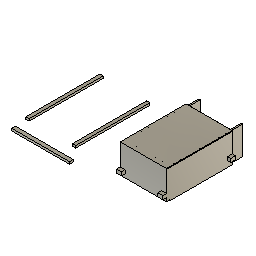
USV_cover_rect v23 (Autodesk Fusion 360 design; units mm, degrees)
Autodesk Fusion 360 part; units mm, degrees
note: some values were not read from the file. Chosen so that the rebuilt part matches the saved one: which face or edge a step refers to.
box "Primitiva de caixa1" add length 8 width 112 height 200 placed x (0, 1, 0) y (-1, 0, 0) z (0, 0, 1) at (112, 0, 0) makes body 1
box "Primitiva de caixa2" add length 100 width 3 height 200 placed x (0, 1, 0) y (-1, 0, 0) z (0, 0, 1) at (112, 0, 0) bodies 1
extrude "Extrusão1" cut 1 faces at (73.6667, 2.6667, 200) along direction (0, 0, -1) blind 100 on bodies 1 bodies 1
box "Primitiva de caixa3" add length 100 width 3 height 100 placed x (0, 1, 0) y (-1, 0, 0) z (0, 0, 1) at (3, 0, 0) bodies 1
box "Primitiva de caixa4" cut length 5 width 112 height -5 placed x (0, 1, 0) y (-1, 0, 0) z (0, 0, 1) at (112, 0, 0) bodies 1
box "Primitiva de caixa5" cut length 5 width 112 height 1 placed x (0, 1, 0) y (-1, 0, 0) z (0, 0, 1) at (112, 0, 0) bodies 1
box "Primitiva de caixa6" add length 5 width 110 height 5 placed x (0, -1, 0) y (1, 0, 0) z (0, 0, 1) at (0.5, 0, 0) bodies 1
delete_face "DeleteFace1" 6 faces at (73.8333, 0, 0.6667) (0.5, -3.3333, 2) (110.5, -3.3333, 2) (73.8333, -1.6667, 0) (73.8333, -5, 3.3333) (73.8333, -1.6667, 5) on bodies 1
box "Primitiva de caixa7" cut length 5 width 109 height 2 placed x (0, 1, 0) y (-1, 0, 0) z (0, 0, 1) at (110.5, 0, 0) bodies 1
box "Primitiva de caixa9" add length 1 width 1.5 height 109 placed x (0, 0, -1) y (0, -1, 0) z (-1, 0, 0) at (110.5, 1.5, 2) bodies 1
move_face "Deslocar faces1" offset -90 1 faces at (38.3333, 2.6667, 100) on bodies 1
sketch "Esboço10" plane through (0, 0, 0) normal (0, 0, 1) x (1, 0, 0)
sketch "Esboço11" plane through (0, 0, 0) normal (0, 0, 1) x (1, 0, 0)
box "Primitiva de caixa10" add length 10 width 3.49 height 10 placed x (0, 1, 0) y (-1, 0, 0) z (0, 0, 1) at (6.49, 95, 0) bodies 1
box "Primitiva de caixa11" add length 10 width 3.49 height 10 placed x (0, 1, 0) y (-1, 0, 0) z (0, 0, 1) at (109, 95, 0) bodies 1
extrude "Extrusão2" add 1 faces at (38.3333, 2.6667, 10) along direction (0, 0, 1) blind 60 on bodies 1 bodies 1
move_face "Deslocar faces2" offset 60 2 faces at (107.8367, 105, 23.3333) (110, 100, 46.6667) on bodies 1
move_face "Deslocar faces3" offset -60 1 faces at (106.6733, 95, 46.6667) on bodies 1
move_face "Deslocar faces4" offset 60 2 faces at (2, 100, 46.6667) (4.1633, 105, 46.6667) on bodies 1
move_face "Deslocar faces5" offset -60 1 faces at (5.3267, 95, 23.3333) on bodies 1
extrude "Extrusão3" add 2 faces at (107.8367, 165, 23.3333) (5.3267, 165, 23.3333) along direction (0, 1, 0) blind 20 on bodies 1 bodies 1
box "Primitiva de caixa12" add length 3.5 width 4 height 3.5 placed x (0, 0, 1) y (-1, 0, 0) z (0, -1, 0) at (112, 0, 6.5) bodies 1
extrude "Extrusão4" add 1 faces at (110.6667, -1.1667, 6.5) along direction (0, 0, -1) blind 0.5 on bodies 1 bodies 1
extrude "Extrusão5" add 1 faces at (108, -1.1667, 8.6667) along direction (-1, 0, 0) blind 2 on bodies 1 bodies 1
box "Primitiva de caixa13" add length 8.5 width 21 height -6 placed x (0, 0, -1) y (-1, 0, 0) z (0, 1, 0) at (21, 0, 19.5) bodies 1
extrude "Extrusão6" add 1 faces at (14, -4, 11) along direction (0, 0, 1) blind 6 on bodies 1 bodies 1
extrude "Extrusão7" cut 1 faces at (14, -4, 19.5) along direction (0, 0, 1) blind 6 on bodies 1 bodies 1
extrude "Extrusão8" cut 1 faces at (21, -4, 13.8333) along direction (-1, 0, 0) blind 9.3 on bodies 1 bodies 1
extrude "Extrusão9" add 1 faces at (108, -3.5, 7.3333) along direction (0, -1, 0) blind 2.5 on bodies 1 bodies 1
box "Primitiva de caixa14" add length 12 width 13 height 6 placed x (0, 0, 1) y (0, -1, 0) z (1, 0, 0) at (112, 160, 5) bodies 1
extrude "Extrusão10" cut 1 faces at (114, 147, 13) along direction (0, 1, 0) blind 7 on bodies 1 bodies 1
extrude "Extrusão11" cut 1 faces at (114, 158, 17) along direction (0, 0, -1) blind 8 on bodies 1 bodies 1
box "Primitiva de caixa15" add length 4 width 6 height 6 placed x (0, 0, 1) y (0, 1, 0) z (-1, 0, 0) at (0, 154, 5) bodies 1
sketch "Esboço22" plane through (112, 0, 0) normal (1, 0, 0) x (0, 1, 0)
  line L0 (160, 5) -> (154, 5)
  line L1 (154, 5) -> (154, 9)
  line L2 (154, 9) -> (160, 9)
  line L3 (160, 9) -> (160, 70)
  line L4 (160, 70) -> (0, 70)
  line L5 (0, 70) -> (0, 10)
  line L6 (0, 10) -> (-6, 10)
  line L7 (-6, 10) -> (-6, 6)
  line L8 (-6, 6) -> (0, 6)
  line L9 (0, 6) -> (0, 1)
  line L10 (0, 1) -> (5, 1)
  line L11 (5, 1) -> (5, 0)
  line L12 (5, 0) -> (160, 0)
  line L13 (160, 0) -> (160, 5)
box "Primitiva de caixa20" add length 52 width 160 height 6.5 placed x (0, 0, -1) y (0, 1, 0) z (1, 0, 0) at (112, 0, 70) bodies 1
sketch "Esboço24" plane through (0, 0, 70) normal (0, 0, 1) x (-1, 0, 0)
  line L0 (-109, -160) -> (-109, -185)
  line L1 (-109, -185) -> (-105.51, -185)
  line L2 (-105.51, -185) -> (-105.51, -155)
  line L3 (-105.51, -155) -> (-109, -155)
  line L4 (-109, -155) -> (-109, -8)
  line L5 (-109, -8) -> (-3, -8)
  line L6 (-3, -8) -> (-3, -155)
  line L7 (-3, -155) -> (-6.49, -155)
  line L8 (-6.49, -155) -> (-6.49, -185)
  line L9 (-6.49, -185) -> (-3, -185)
  line L10 (-3, -185) -> (-3, -160)
  line L11 (-3, -160) -> (0, -160)
box "Primitiva de caixa21" add length 3 width 9 height 1 placed x (0, -1, 0) y (1, 0, 0) z (0, 0, 1) at (109, 8, 70) bodies 1
extrude "Extrusão14" cut 1 faces at (115, 7, 71) along direction (0, 0, -1) blind 1 on bodies 1 bodies 1
box "Primitiva de caixa22" add length 4 width 3 height 1 placed x (0, -1, 0) y (1, 0, 0) z (0, 0, 1) at (109, 8, 70) bodies 1
box "Primitiva de caixa23" cut length 147 width 2.5 height -61 placed x (0, 1, 0) y (-1, 0, 0) z (0, 0, 1) at (114.5, 8, 70) bodies 1
extrude "Extrusão15" cut 1 faces at (118.5, 106.6667, 52.6667) along direction (-1, 0, 0) blind 6.5 on bodies 1 bodies 1
box "Primitiva de caixa24" add length 52 width 160 height -2 placed x (0, 0, -1) y (0, -1, 0) z (-1, 0, 0) at (0, 160, 70) bodies 1
move_face "MoverFace1" by (-26.3793, 1.2468, -0.5389) 1 faces at (111, 6.6667, 71) on bodies 1
extrude "Extrusão16" add 1 faces at (111, 6.6667, 70.4611) along direction (0, 0, 1) blind 2 on bodies 1 bodies 1
extrude "Extrusão17" add 1 faces at (109, 5.3333, 71.6407) along direction (-1, 0, 0) blind 109 on bodies 1 bodies 1
box "Primitiva de caixa25" cut length 147 width 2.5 height -61 placed x (0, -1, 0) y (1, 0, 0) z (0, 0, 1) at (-2.5, 155, 70) bodies 1
extrude "Extrusão18" cut 1 faces at (74.6667, 4, 70.8204) along direction (0, 1, 0) blind 4 on bodies 1 bodies 1
box "Primitiva de caixa26" add length 3 width 2 height -1 placed x (0, -1, 0) y (1, 0, 0) z (0, 0, 1) at (109, 8, 70) bodies 1
box "Primitiva de caixa27" cut length 2.5 width 106 height -52 placed x (0, -1, 0) y (1, 0, 0) z (0, 0, 1) at (3, 5, 70) bodies 1
extrude "Extrusão25" cut 1 faces at (110, 160, 29.3333) along direction (0, -1, 0) blind 3.3 on bodies 1 bodies 1
extrude "Extrusão26" cut 1 faces at (2, 160, 26.3333) along direction (0, -1, 0) blind 3.3 on bodies 1 bodies 1
extrude "Extrusão27" add 1 faces at (-2, 154, 7.6667) along direction (0, -1, 0) blind 9 on bodies 1 bodies 1
extrude "Extrusão28" add 1 faces at (114, 154, 7.6667) along direction (0, -1, 0) blind 9 on bodies 1 bodies 1
delete_face "DeleteFace2" 1 faces at (109, 3.3333, 35.3333) on bodies 1
box "Primitiva de caixa34" cut length 30 width 3.49 height -0.01 placed x (0, 1, 0) y (-1, 0, 0) z (0, 0, 1) at (109, 155, 70) bodies 1
box "Primitiva de caixa35" cut length 30 width 3.49 height -0.01 placed x (0, -1, 0) y (1, 0, 0) z (0, 0, 1) at (3, 185, 70) bodies 1
box "Primitiva de caixa36" cut length 30 width 3.49 height 0.01 placed x (0, 1, 0) y (-1, 0, 0) z (0, 0, 1) at (6.49, 155, 69.99) bodies 1
sketch "Esboço41" plane through (0, 0, 70) normal (0, 0, 1) x (-1, 0, 0)
  line L0 (-3, -8) -> (-3, -156.7)
  line L1 (-3, -156.7) -> (0, -156.7)
  line L2 (0, -156.7) -> (0, 0)
  line L3 (0, 0) -> (-112, 0)
  line L4 (-112, 0) -> (-112, -156.7)
  line L5 (-112, -156.7) -> (-109, -156.7)
  line L6 (-109, -156.7) -> (-109, -8)
  line L7 (-109, -8) -> (-3, -8)
box "Primitiva de caixa37" add length 185 width 265 height 2 placed x (0, 1, 0) y (-1, 0, 0) z (0, 0, 1) at (265, 0, 70) bodies 1
box "Primitiva de caixa38" add length 190 width 153 height 0.5 placed x (0, -1, 0) y (1, 0, 0) z (0, 0, 1) at (-153, 185, 72) separate body makes body 2
move_face "Deslocar faces6" offset 2 1 faces at (-102, 121.6667, 72) on bodies 2
extrude "Extrusão29" cut 1 faces at (-102, 121.6667, 72.5) along direction (0, 0, -1) blind 0.5 on bodies 2 bodies 2
extrude "Extrusão30" cut 1 faces at (-51, -5, 70.6667) along direction (0, 1, 0) blind 5 on bodies 2 bodies 2
box "Primitiva de caixa39" add length 165 width 418 height -2 placed x (0, -1, 0) y (1, 0, 0) z (0, 0, 1) at (-153, 0, 72) bodies 1 2
extrude "Extrusão31" cut 2 faces at (-153, -110, 70.6667) (-153, 61.6667, 70.6667) along direction (1, 0, 0) blind 150 on bodies 1 bodies 1
extrude "Extrusão32" cut 1 faces at (175.6667, -165, 70.6667) along direction (0, 1, 0) blind 95 on bodies 1 bodies 1
extrude "Extrusão33" cut 1 faces at (175.6667, -70, 70.6667) along direction (0, 1, 0) blind 65 on bodies 1 bodies 1
extrude "Extrusão34" cut 2 faces at (265, -3.3333, 70.6667) (265, 123.3333, 70.6667) along direction (-1, 0, 0) blind 150 on bodies 1 bodies 1
extrude "Extrusão35" add 2 faces at (115, 123.3333, 70.6667) (115, -3.3333, 70.6667) along direction (1, 0, 0) blind 0.441 on bodies 1 bodies 1
extrude "Extrusão36" add 2 faces at (115.441, -3.3333, 70.6667) (115.441, 123.3333, 70.6667) along direction (1, 0, 0) blind 2 on bodies 1 bodies 1
extrude "Extrusão37" add 2 faces at (117.441, 123.3333, 70.6667) (117.441, -3.3333, 70.6667) along direction (1, 0, 0) blind 2 on bodies 1 bodies 1
extrude "Extrusão38" cut 2 faces at (-3, 61.6667, 70.6667) (-3, -3.3333, 70.6667) along direction (1, 0, 0) blind 3 on bodies 1 bodies 1
extrude "Extrusão39" cut 2 faces at (119.441, 123.3333, 70.6667) (119.441, -3.3333, 70.6667) along direction (-1, 0, 0) blind 7 on bodies 1 bodies 1
extrude "Extrusão40" cut 1 faces at (112.441, -3.3333, 70.6667) along direction (1, 0, 0) blind 1 on bodies 1 bodies 1
extrude "Extrusão41" cut 2 faces at (112.441, 123.3333, 70.6667) (112.441, -3.3333, 70.6667) along direction (-1, 0, 0) blind 0.5 on bodies 1 bodies 1
extrude "Extrusão42" cut 1 faces at (37.3137, -5, 70.6667) along direction (0, 1, 0) blind 5 on bodies 1 bodies 1
box "Primitiva de caixa40" add length 2 width 185 height 0.057 placed x (0, 0, 1) y (0, -1, 0) z (1, 0, 0) at (111.941, 185, 70) bodies 1
box "Primitiva de caixa41" cut length 1.502 width 30 height -2 placed x (0, 0, -1) y (0, 1, 0) z (1, 0, 0) at (6.49, 155, 1.5025) bodies 1
extrude "Extrusão43" cut 1 faces at (4.49, 175, 1.0018) along direction (0, 0, -1) blind 1 on bodies 1 bodies 1
box "Primitiva de caixa42" cut length 1.5 width 30 height -3.5 placed x (0, 0, 1) y (0, 1, 0) z (-1, 0, 0) at (105.51, 155, 0) bodies 1
extrude "Extrusão44" cut 1 faces at (5.1567, 165, 1.5025) along direction (0, 0, 1) blind 0.02 on bodies 1 bodies 1
extrude "Extrusão45" add 1 faces at (5.1567, 165, 1.5225) along direction (0, 0, -1) blind 0.022 on bodies 1 bodies 1
move_face "Deslocar faces7" offset -28.3 1 faces at (37.3327, 185, 71.3333) on bodies 1
move_face "Deslocar faces8" offset -1.5 1 faces at (4.49, 165, 1.0003) on bodies 1
move_face "Deslocar faces9" offset 9.5 1 faces at (116, 149.5667, 9) on bodies 1
move_face "Deslocar faces10" offset -9.5 1 faces at (114, 152.8, 5) on bodies 1
move_face "Deslocar faces11" offset 4.5 1 faces at (116, 149.5667, 18.5) on bodies 1
move_face "Deslocar faces12" offset 2 1 faces at (118, 148.9, 17.3333) on bodies 1
move_face "Deslocar faces13" offset 9.5 1 faces at (-2, 148.9, 9) on bodies 1
move_face "Deslocar faces14" offset -9.5 1 faces at (-4, 148.9, 5) on bodies 1
move_face "Deslocar faces15" offset 2 1 faces at (-2, 148.9, 18.5) on bodies 1
move_face "Deslocar faces16" offset 2.5 1 faces at (-2, 148.9, 20.5) on bodies 1
move_face "Deslocar faces17" offset 2 1 faces at (-6, 148.9, 17.3333) on bodies 1
move_face "Deslocar faces18" offset 3 1 faces at (76.566, 0, 33.1667) on bodies 1
move_face "Deslocar faces19" offset -1 1 faces at (37.8333, -1.5, 1) on bodies 1
move_face "Deslocar faces20" offset 6 1 faces at (110, -5, 10) on bodies 1
move_face "Deslocar faces21" offset -6 1 faces at (110, -5, 6) on bodies 1
extrude "Extrusão46" add 1 faces at (110, -5, 12) along direction (0, 0, -1) blind 1 on bodies 1 bodies 1
move_face "Deslocar faces22" offset 5.7 1 faces at (106, -4, 14.3333) on bodies 1
move_face "Deslocar faces23" offset 6 1 faces at (7.8, -6, 13.8333) on bodies 1
move_face "Deslocar faces24" offset 6 1 faces at (104.2, -6, 13) on bodies 1
move_face "Deslocar faces25" offset 3.5 1 faces at (108.1, -9, 16) on bodies 1
box "Primitiva de caixa43" add length 180 width 8 height 5.3 placed x (0, -1, 0) y (1, 0, 0) z (0, 0, 1) at (-118, 170, 0) separate body makes body 3
move_body "Mover3" bodies 3 to x (1, 0, 0) y (0, 1, 0) z (0, 0, 1) at (-0.5021, 9.3986, 2.4431)
copy_body "Copiar e colar corpos1" bodies 3 makes body 4
copy_body "Copiar e colar corpos2" bodies 3 makes body 5
move_body "Mover4" bodies 5 to x (1, 0, 0) y (0, 1, 0) z (0, 0, 1) at (-113, 0, 0)
box "Primitiva de caixa45" add length 9 width 140 height 5.5 placed x (0, -1, 0) y (1, 0, 0) z (0, 0, 1) at (-220, -250, 70) separate body makes body 6
move_body "Mover5" bodies 6 to x (1, 0, 0) y (0, 1, 0) z (0, 0, 1) at (10.3025, 217.0839, -53.2186)
move_body "Mover6" bodies 6 to x (1, 0, 0) y (0, 1, 0) z (0, 0, 1) at (-14.6765, 0, -14.5116)
